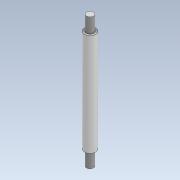
# Autodesk Inventor part: Eje Biela
Saved by Autodesk Inventor 2021 (Build 250183000, 183)
## iProperties
Created: 2021-06-19
Part Number: Eje Biela
Material: Generic
Document SubType Name: Modeling
Designer: Andrés Holguín
Density: 1 g/cm^3
Appearance: Default
Author: Andrés Holguín
Autodesk Inventor part; units mm, degrees
ref_plane "YZ Plane" through (0, 0, 0) normal (1, 0, 0) x (0, 1, 0)
ref_plane "XZ Plane" through (0, 0, 0) normal (0, 1, 0) x (-1, 0, 0)
ref_plane "XY Plane" through (0, 0, 0) normal (0, 0, 1) x (1, 0, 0)
sketch "Sketch1" plane through (0, 0, 0) normal (0, 1, 0) x (-1, 0, 0)
  circle A0 centre (0, 0) radius 15
  dimension "d7" = 30
  constraints: 1 centre point, 1 coincident
  measures "d7" diameter of A0
extrude "Extrusion1" add sketch "Sketch1" along normal mid plane 176.675
sketch "Sketch2" plane through (0, 88.3375, 0) normal (0, 1, 0) x (1, 0, 0)
  circle A0 centre (0, 0) radius 9.525
  circle A1 centre (0, 0) radius 15 projected
  circle A2 centre (0, 0) radius 15
  dimension "d6" = 19.05
  constraints: 2 centre point, 2 coincident, 1 concentric
  measures "d6" diameter of A0
extrude "Extrusion2" cut sketch "Sketch2" against normal blind 39.7
fillet "Fillet1" radius 0.5 1 edges at (-9.525, 48.6375, 0)
thread "Thread3" size "M20x0.75" class "6g" standard "ANSI Metric M Profile" length 44.7802
mirror "Mirror2" about plane through (0, -88.3375, 0) normal (0, -1, 0) of "Extrusion2", "Extrusion1", "Fillet1"
body "Solid1"
